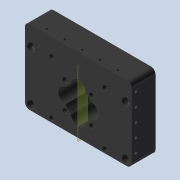
# Autodesk Inventor part: Nikon_Ti2E
Saved by Autodesk Inventor 2022 (Build 260153000, 153)
## iProperties
Created: 2021-06-08
Part Number: Nikon_Ti2E
Material: Generic
Document SubType Name: Modeling
Designer: wanghaoran
Density: 1 g/cm^3
Appearance: Default
Author: wanghaoran
Autodesk Inventor part; units mm, degrees
ref_plane "YZ Plane" through (0, 0, 0) normal (1, 0, 0) x (0, 1, 0)
ref_plane "XZ Plane" through (0, 0, 0) normal (0, 1, 0) x (-1, 0, 0)
ref_plane "XY Plane" through (0, 0, 0) normal (0, 0, 1) x (1, 0, 0)
sketch "Sketch1" plane through (0, 0, 0) normal (0, 0, 1) x (1, 0, 0)
  line L0 (0, 0) -> (120, 0)
  line L1 (120, 0) -> (120, 68)
  line L2 (120, 68) -> (0, 68)
  line L3 (0, 68) -> (0, 0)
  dimension "d0" = 120
  dimension "d1" = 68
  constraints: 8 end point, 2 parallel, 1 horizontal, 1 perpendicular
  measures "d0" distance of L2.end L1.end
  measures "d1" distance of L1.end L0.end
extrude "Extrusion1" add sketch "Sketch1" along normal blind 10
sketch "Sketch2" plane through (0, 0, 10) normal (0, 0, 1) x (1, 0, 0)
  circle A0 centre (6.6, 6) radius 2.9
  line L0 (0, 0) -> (120, 0) projected
  line L1 (0, 68) -> (0, 0) projected
  circle A1 centre (113.4, 6) radius 2.9
  circle A2 centre (6.6, 62) radius 2.9
  circle A3 centre (113.4, 62) radius 2.9
  circle A4 centre (60, 34) radius 17
  circle A5 centre (45, 49) radius 3.25
  circle A6 centre (75, 49) radius 3.25
  circle A7 centre (45, 19) radius 3.25
  circle A8 centre (75, 19) radius 3.25
  line L2 (120, 68) -> (0, 68) projected
  circle A9 centre (60, 48.4582) radius 8.4721
  circle A10 centre (45.5418, 34) radius 8.4721
  circle A11 centre (60, 19.5418) radius 8.4721
  circle A12 centre (74.4582, 34) radius 8.4721
  point P0 (68.4673, 19.2587)
  point P1 (51.5327, 19.2587)
  point P2 (74.7413, 25.5327)
  point P3 (74.7413, 42.4673)
  point P4 (45.2587, 25.5327)
  point P5 (45.2587, 42.4673)
  point P6 (51.5327, 48.7413)
  point P7 (68.4673, 48.7413)
  dimension "d4" = 5.8
  dimension "d5" = 6
  dimension "d6" = 6.6
  dimension "d9" = 106.8
  dimension "d12" = 56
  dimension "d15" = 34
  dimension "d16" = 6.5
  dimension "d17" = 15
  dimension "d18" = 15
  dimension "d19" = 34
  dimension "d20" = 60
  dimension "d23" = 30
  dimension "d26" = 30
  dimension "d82" = 360
  constraints: 13 centre point, 2 horizontal, 2 vertical, 21 other
  measures "d4" diameter of A0
  measures "d5" distance from line of L0 A0.centre
  measures "d6" distance from line of L1 A0.centre
  measures "d9" distance of A0.centre A1.centre
  measures "d12" distance of A0.centre A2.centre
  measures "d15" diameter of A4
  measures "d16" diameter of A5
  measures "d17" horizontal distance of A5.centre A4.centre
  measures "d18" horizontal distance of A4.centre A5.centre
  measures "d19" distance from line of L0 A4.centre
  measures "d20" distance from line of L1 A4.centre
  measures "d23" distance of A5.centre A6.centre
  measures "d26" distance of A5.centre A7.centre
extrude "Extrusion2" cut sketch "Sketch2" against normal through all contours A0 | A1 | A2 | A3 | A4 A12 | A4 A12 | A12 A4 A11 A10 A9 | A9 A4 | A4 A9 | A11 A4 | A4 A11 | A10 A4 | A4 A10
ref_plane "Work Plane1" through (60, 0, 0) normal (1, 0, 0) x (0, 0, -1)
ref_plane "Arbeitsebene2" through (60, 0, 0) normal (-1, 0, 0) x (0, 0, 1)
sketch "Sketch5" plane through (0, 0, 10) normal (0, 0, 1) x (1, 0, 0)
  circle A0 centre (45, 49) radius 1.35
  circle A1 centre (60, 34) radius 17 projected
  line L0 (45, 49) -> (49.5107, 49)
  line L1 (49.5107, 49) -> (49.5107, 56.375)
  circle A2 centre (75, 49) radius 1.35
  circle A3 centre (45, 19) radius 1.35
  circle A4 centre (75, 19) radius 1.35
  circle A5 centre (30, 64) radius 1.35
  circle A6 centre (90, 64) radius 1.35
  circle A7 centre (30, 4) radius 1.35
  circle A8 centre (90, 4) radius 1.35
  point P0 (0, 0)
  dimension "d43" = 2.7
  dimension "d45" = 15
  dimension "d46" = 15
  dimension "d49" = 30
  dimension "d52" = 30
  dimension "d62" = 2.7
  dimension "d63" = 30
  dimension "d64" = 30
  dimension "d67" = 60
  dimension "d70" = 60
  constraints: 8 centre point, 4 end point, 3 horizontal, 2 vertical, 1 perpendicular, 12 other
  measures "d43" diameter of A0
  measures "d45" horizontal distance of A1.centre L0.start
  measures "d46" horizontal distance of L0.start A1.centre
  measures "d49" distance of L0.start A2.centre
  measures "d52" distance of L0.start A3.centre
  measures "d62" diameter of A5
  measures "d63" horizontal distance of A5.centre A1.centre
  measures "d64" horizontal distance of A5.centre A1.centre
  measures "d67" distance of A5.centre A6.centre
  measures "d70" distance of A5.centre A7.centre
hole "Hole1" at (75, 49, 10) at (75, 19, 10) at (45, 19, 10) at (45, 49, 10) at (30, 64, 10) at (90, 64, 10) at (90, 4, 10) at (30, 4, 10) direction (0, 0, -1) diameter 2.8 end through all counterbore diameter 6.1 counterbore depth 9.5
sketch "Sketch8" plane through (0, 0, 0) normal (0, 0, -1) x (-1, 0, 0)
  circle A0 centre (-90, 4) radius 1.4 projected
  circle A1 centre (-30, 64) radius 1.4 projected
  circle A2 centre (-45, 19) radius 1.4 projected
  circle A3 centre (-75, 49) radius 1.4 projected
  circle A4 centre (-75, 19) radius 1.4 projected
  circle A5 centre (-45, 49) radius 1.4 projected
  circle A6 centre (-90, 64) radius 1.4 projected
  circle A7 centre (-30, 4) radius 1.4 projected
  circle A8 centre (-113.4, 62) radius 2.9 projected
  circle A9 centre (-113.4, 6) radius 2.9 projected
  circle A10 centre (-6.6, 6) radius 2.9 projected
  circle A11 centre (-6.6, 62) radius 2.9 projected
  arc A12 (-51.5327, 48.7413) -> (-68.4673, 48.7413) centre (-60, 48.4582) ccw projected
  arc A13 (-45.2587, 42.4673) -> (-51.5327, 48.7413) centre (-60, 34) ccw projected
  arc A14 (-45.2587, 25.5327) -> (-45.2587, 42.4673) centre (-45.5418, 34) ccw projected
  arc A15 (-51.5327, 19.2587) -> (-45.2587, 25.5327) centre (-60, 34) ccw projected
  arc A16 (-68.4673, 19.2587) -> (-51.5327, 19.2587) centre (-60, 19.5418) ccw projected
  arc A17 (-74.7413, 25.5327) -> (-68.4673, 19.2587) centre (-60, 34) ccw projected
  arc A18 (-74.7413, 42.4673) -> (-74.7413, 25.5327) centre (-74.4582, 34) ccw projected
  arc A19 (-68.4673, 48.7413) -> (-74.7413, 42.4673) centre (-60, 34) ccw projected
  line L0 (0, 68) -> (0, 0) projected
  line L1 (-120, 68) -> (0, 68) projected
  line L2 (-120, 0) -> (-120, 68) projected
  line L3 (0, 0) -> (-120, 0) projected
extrude "Extrusion5" add sketch "Sketch8" along normal blind 17
sketch "Sketch9" plane through (0, 0, -17) normal (0, 0, -1) x (-1, 0, 0)
  circle A0 centre (-75, 19) radius 1.4 projected
  circle A1 centre (-45, 19) radius 1.4 projected
  circle A2 centre (-45, 49) radius 1.4 projected
  circle A3 centre (-75, 49) radius 1.4 projected
  circle A4 centre (-75, 19) radius 2.55
  circle A5 centre (-75, 49) radius 1.4 projected
  circle A6 centre (-75, 49) radius 2.55
  circle A7 centre (-45, 49) radius 1.4 projected
  circle A8 centre (-45, 49) radius 2.55
  circle A9 centre (-45, 19) radius 2.55
  circle A10 centre (-90, 64) radius 1.4 projected
  circle A11 centre (-90, 64) radius 2.55
  circle A12 centre (-90, 64) radius 3.05 projected
  line L0 (-90, 64) -> (-85.596, 64)
  line L1 (-85.596, 64) -> (-85.596, 65.4)
  line L2 (-87.2903, 65.4) -> (-82.8137, 65.4) projected
  circle A13 centre (-30, 64) radius 2.55
  circle A14 centre (-90, 4) radius 2.55
  circle A15 centre (-30, 4) radius 2.55
  point P0 (0, 0)
  dimension "d99" = 5.1
  dimension "d100" = 5.1
  dimension "d101" = 5.1
  dimension "d102" = 5.1
  dimension "d113" = 5.1
  dimension "d116" = 60
  dimension "d119" = 60
  constraints: 8 centre point, 5 coincident, 4 end point, 2 horizontal, 1 perpendicular, 1 point on line, 1 vertical, 6 other
  measures "d99" diameter of A4
  measures "d100" diameter of A6
  measures "d101" diameter of A8
  measures "d102" diameter of A9
  measures "d113" diameter of A11
  measures "d116" distance of A11.centre A13.centre
  measures "d119" distance of A11.centre A14.centre
extrude "Extrusion7" cut sketch "Sketch9" against normal blind 12.4 contours A0 | A1 | A2 | A3 | A4 | A6 | A8 | A9 | A10 | A11 | A12 | A13 | A14 | A15
sketch "Sketch10" plane through (0, 0, 10) normal (0, 0, 1) x (1, 0, 0)
  circle A0 centre (6.6, 6) radius 2.9 projected
  circle A1 centre (6.6, 6) radius 4.7
  circle A2 centre (6.6, 62) radius 2.9 projected
  circle A3 centre (6.6, 62) radius 4.7
  circle A4 centre (113.4, 62) radius 2.9 projected
  circle A5 centre (113.4, 62) radius 4.7
  circle A6 centre (113.4, 6) radius 2.9 projected
  circle A7 centre (113.4, 6) radius 4.7
  point P0 (0, 0)
  dimension "d107" = 9.4
  dimension "d108" = 9.4
  dimension "d109" = 9.4
  dimension "d110" = 9.4
  constraints: 4 centre point, 4 coincident
  measures "d107" diameter of A1
  measures "d108" diameter of A3
  measures "d109" diameter of A5
  measures "d110" diameter of A7
extrude "Extrusion8" cut sketch "Sketch10" against normal blind 22.4 contours A0 | A1 | A2 | A3 | A4 | A5 | A6 | A7
sketch "Sketch11" plane through (0, 68, 10) normal (0, 1, 0) x (1, 0, 0)
  line L0 (120, 27) -> (120, 0) projected
  line L1 (0, 27) -> (0, 0) projected
  line L2 (120, 0) -> (0, 0) projected
  line L3 (120, 27) -> (120, 0) projected
  line L4 (0, 27) -> (120, 27) projected
  circle A0 centre (100, 5) radius 1.4
  circle A1 centre (80, 5) radius 1.4
  circle A2 centre (60, 5) radius 1.4
  circle A3 centre (40, 5) radius 1.4
  circle A4 centre (20, 5) radius 1.4
  point P0 (0, 10)
  dimension "d122" = 2.8
  dimension "d123" = 5
  dimension "d124" = 20
  dimension "d127" = 20
  constraints: 5 centre point, 1 horizontal, 8 other
  measures "d122" diameter of A0
  measures "d123" distance from line of L2 A0.centre
  measures "d124" distance from line of L0 A0.centre
  measures "d127" distance of A0.centre A1.centre
extrude "Extrusion9" add sketch "Sketch11" along normal blind 15.7
sketch "Sketch12" plane through (0, 0, -17) normal (-1, 0, 0) x (0, 0, 1)
  circle A0 centre (22, 72.5) radius 1.4
  line L0 (27, 0) -> (27, 83.7) projected
  line L1 (0, 83.7) -> (27, 83.7) projected
  circle A1 centre (22, 57.5) radius 1.4
  circle A2 centre (22, 42.5) radius 1.4
  circle A3 centre (22, 27.5) radius 1.4
  circle A4 centre (22, 12.5) radius 1.4
  point P0 (17, 0)
  dimension "d134" = 2.8
  dimension "d135" = 5
  dimension "d136" = 11.2
  dimension "d139" = 15
  constraints: 5 centre point, 1 vertical, 8 other
  measures "d134" diameter of A0
  measures "d135" distance from line of L0 A0.centre
  measures "d136" distance from line of L1 A0.centre
  measures "d139" distance of A0.centre A1.centre
extrude "Extrusion10" cut sketch "Sketch12" against normal blind 10
mirror "Mirror1" about plane through (60, 0, 0) normal (-1, 0, 0) of "Extrusion10"
fillet "Fillet2" radius 5 4 edges at (0, 83.7, -3.5) (120, 83.7, -3.5) (0, 0, -3.5) (120, 0, -3.5)
body "Solid1"
